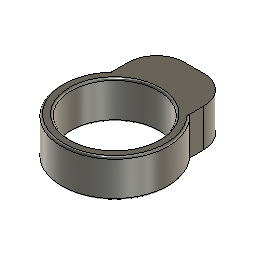
ring (Autodesk Fusion 360 design; units mm, degrees)
Autodesk Fusion 360 part; units mm, degrees
note: some values were not read from the file. Set by a fixed rule: which sketch regions a step uses.
sketch "Esboço1" plane through (0, 0, 0) normal (0, 0, 1) x (1, 0, 0)
  circle A0 centre (0, 0) radius 11.5
  circle A1 centre (0, 0) radius 14
  line L0 (-10, 9.798) -> (-10, 21)
  line L1 (-10, 21) -> (10, 21)
  line L2 (10, 21) -> (10, 9.798)
  line L3 (0, 0) -> (0, 14)
  dimension "d1" = 23
  dimension "d2" = 28
  dimension "d3" = 20
  dimension "d5" = 7
  constraint coincident A0.centre A1.centre
  constraint coincident A1 L0.start
  constraint vertical L0
  constraint perpendicular L0 L1
  constraint coincident A1 L2.end
  constraint perpendicular L1 L2
  constraint coincident A1 L3.end
  constraint vertical L3
  measures "d1" diameter of A0
  measures "d2" diameter of A1
  measures "d3" distance of L0 L2
  measures "d5" distance of L1 L3.end
extrude "Extrusão1" add sketch "Esboço1" along normal blind 10
hole "Furo1" at (0, 21, 5) direction (0, -1, 0) diameter 2.8 depth 5.5 tip angle 180
fillet "Arredondamento1" radius 0.5 4 edges at (-10.7218, 4.1586, 10) (-10.7218, 4.1586, 0) (0, -14, 0) (0, -14, 10)
fillet "Arredondamento2" radius 7.5 2 edges at (-10, 21, 5) (10, 21, 5)
